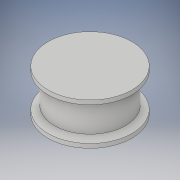
# Autodesk Inventor part: Felge_V1
Saved by Autodesk Inventor 2017.3 (Build 213257000, 257)
## iProperties
Part Number: Felge_V1
Material: Generisch
Document SubType Name: Modeling
Designer: Enno-LT
Density: 1 g/cm^3
Appearance: Vorgabe
Author: Enno-LT
Autodesk Inventor part; units mm, degrees
ref_plane "YZ Plane" through (0, 0, 0) normal (1, 0, 0) x (0, 1, 0)
ref_plane "XZ Plane" through (0, 0, 0) normal (0, 1, 0) x (-1, 0, 0)
ref_plane "XY Plane" through (0, 0, 0) normal (0, 0, 1) x (1, 0, 0)
sketch "Skizze1" plane through (0, 0, 0) normal (0, 0, 1) x (1, 0, 0)
  circle A0 centre (0, 0) radius 20
  dimension "d0" = 40
  constraints: 1 centre point, 1 coincident
  measures "d0" diameter of A0
extrude "Extrusion1" add sketch "Skizze1" along normal mid plane 20
sketch "Skizze2" plane through (0, 0, 0) normal (1, 0, 0) x (0, 1, 0)
  line L0 (20, -10) -> (20, 10) projected
  line L1 (20, 8) -> (20, -8)
  line L2 (17, -6.2679) -> (17, 6.2679)
  line L3 (17, 6.2679) -> (20, 8)
  line L4 (17, -6.2679) -> (20, -8)
  line L5 (20, 10) -> (-20, 10) projected
  line L6 (0, 17.0847) -> (0, -27.9432) construction
  point P0 (0, 0)
  dimension "d3" = 3
  dimension "d4" = 2
  dimension "d5" = 2
  dimension "d6" = 60
  dimension "d7" = 60
  constraints: 10 end point, 2 point on line, 2 vertical
  measures "d3" distance between parallel lines of L2 L0
  measures "d4" distance of L0.start L1.end
  measures "d5" distance from line of L5 L1.start
  measures "d6" angle of L0 L3
  measures "d7" angle of L0 L4
revolve "Umdrehung1" cut sketch "Skizze2" angle 360 about axis through (0, 0, 17.0847) along (0, 0, -1)
sketch "Skizze4" plane through (0, 0, 0) normal (1, 0, 0) x (0, 1, 0)
  point P0 (0, 0)
